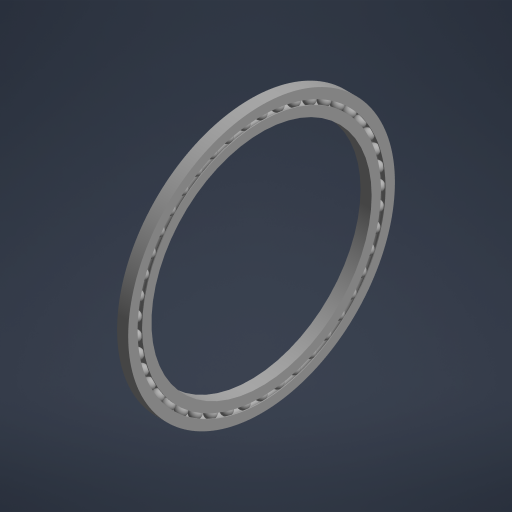
# Autodesk Inventor part: Large bearing
Saved by Autodesk Inventor 2023 (Build 270158000, 158)
## iProperties
Part Number: Large bearing
Material: Generic
Document SubType Name: Modeling
Designer: izack
Appearance: Default
Author: izack
## iProperties of the stored document Large bearing_3DPrint.ipt
Part Number: Large bearing_3DPrint
Material: Generic
Document SubType Name: Modeling
Designer: izack
Appearance: Default
Author: izack
Autodesk Inventor part; units mm, degrees
ref_plane "YZ Plane" through (0, 0, 0) normal (1, 0, 0) x (0, 1, 0)
ref_plane "XZ Plane" through (0, 0, 0) normal (0, 1, 0) x (-1, 0, 0)
ref_plane "XY Plane" through (0, 0, 0) normal (0, 0, 1) x (1, 0, 0)
sketch "Sketch1" plane through (0, 0, 0) normal (0, 1, 0) x (-1, 0, 0)
  line L0 (0, 0) -> (12.958, 0) construction
  line L1 (0, 0) -> (0, -49.6166) construction
  line L2 (0, -49.6166) -> (5, -49.6166)
  line L3 (5, -49.6166) -> (0, -49.6166)
  line L4 (0, -49.6166) -> (0, -52.6166)
  line L5 (5, -52.6166) -> (5, -49.6166)
  circle A0 centre (2.5, -54.8666) radius 2.375
  line L6 (0, -57.1166) -> (0, -60.1166)
  line L7 (0, -60.1166) -> (5, -60.1166)
  line L8 (5, -60.1166) -> (5, -57.1166)
  line L9 (5, -52.6166) -> (0, -52.6166)
  line L10 (5, -57.1166) -> (0, -57.1166)
  line L11 (0, -52.6166) -> (5, -52.6166)
  line L12 (5, -52.6166) -> (5, -53.8666)
  line L13 (5, -53.8666) -> (0, -53.8666)
  line L14 (0, -53.8666) -> (0, -52.6166)
  line L15 (0, -57.1166) -> (5, -57.1166)
  line L16 (5, -57.1166) -> (5, -55.8666)
  line L17 (5, -55.8666) -> (0, -55.8666)
  line L18 (0, -55.8666) -> (0, -57.1166)
  line L19 (4.875, -54.8666) -> (0.125, -54.8666)
  point P0 (4.3414, -56.3666)
  point P1 (0.6586, -56.3666)
  point P2 (0.6586, -53.3666)
  point P3 (4.3414, -53.3666)
  point P4 (1.7397, -57.1166)
  point P5 (3.2603, -57.1166)
  point P6 (1.7397, -52.6166)
  point P7 (3.2603, -52.6166)
  point P8 (4.6542, -53.8666)
  point P9 (0.3458, -53.8666)
  point P10 (4.6542, -55.8666)
  point P11 (0.3458, -55.8666)
  dimension "d0" = 5
  dimension "d2" = 4.75
  dimension "d4" = 49.6166
  dimension "d5" = 3
  dimension "d7" = 5
  dimension "d12" = 3
  dimension "d13" = 2.25
  dimension "d14" = 2.25
  dimension "d15" = 1.25
  dimension "d16" = 1.25
  constraints: 40 end point, 8 horizontal, 6 parallel, 6 point on circle, 3 perpendicular, 2 point on line, 1 centre point, 1 vertical
  measures "d0" distance of L1.end L2.end
  measures "d2" diameter of A0
  measures "d4" distance of L0.start L1.end
  measures "d5" distance of L6.end L6.start
  measures "d7" distance of L6.end L7.end
  measures "d12" distance between parallel lines of L2 L9
  measures "d13" distance from line of A0.centre L10
  measures "d14" distance from line of A0.centre L9
  measures "d15" distance of L11.end L12.end
  measures "d16" distance of L16.end L15.end
revolve "Revolution1" add sketch "Sketch1" angle 360 about axis through (0, 0, 0) along (-1, 0, 0) contours L2 L5 L9 A0 L4 | L9 A0 L13 L14 | L12 L13 A0 L9
revolve "Revolution2" add sketch "Sketch1" angle 360 about axis through (0, 0, 0) along (-1, 0, 0) separate body contours A0 L10 L18 L17 | L17 L16 L10 A0 | A0 L10 L8 L7 L6
revolve "Revolution3" add sketch "Sketch1" angle 360 about axis through (-4.875, 0, -54.8666) along (1, 0, 0) separate body contours L19 A0 L17 | L17 A0 L10 | L10 A0
pattern_circular "Circular Pattern1" count 45 over 360 about axis through (-2.5, 0, 0) along (-1, 0, 0) of "Revolution3" bodies 3
body "Solid1"
body "Solid2"
body "Solid3"
